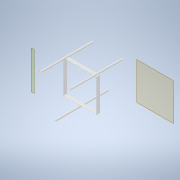
# Autodesk Inventor part: Grid
Saved by Autodesk Inventor 2020 (Build 240168000, 168)
## iProperties
Created: 2022-03-23
Part Number: Grid
Material: Genérico
Document SubType Name: Modeling
Designer: aarco
Density: 1 g/cm^3
Appearance: Valor por defecto
Mass: 1984.02 g
Surface Area: 19686.3 cm^2
Volume: 1984.02 cm^3
Author: aarco
Autodesk Inventor part; units mm, degrees
ref_plane "YZ Plane" through (0, 0, 0) normal (1, 0, 0) x (0, 1, 0)
ref_plane "XZ Plane" through (0, 0, 0) normal (0, 1, 0) x (-1, 0, 0)
ref_plane "XY Plane" through (0, 0, 0) normal (0, 0, 1) x (1, 0, 0)
ref_plane "Plano de trabajo1" through (0, 0, 0) normal (0, 0, 1) x (1, 0, 0)
ref_plane "Plano de trabajo3" through (-2370.6432, -155.0139, 1126.1413) normal (0, 0, -1) x (-1, 0, 0)
sketch "Boceto3" plane through (-2370.6432, -155.0139, 1126.1413) normal (0, 0, -1) x (-1, 0, 0)
  line L0 (-2193.4542, 373.9783) -> (-2193.4542, 1173.9783) projected
  line L1 (-1393.4542, 373.9783) -> (-2193.4542, 373.9783) projected
  line L2 (-1393.4542, 1173.9783) -> (-1393.4542, 373.9783) projected
  line L3 (-2193.4542, 1173.9783) -> (-1393.4542, 1173.9783) projected
  circle A0 centre (-1793.4542, 773.9783) radius 283.4638 projected
  line L4 (-2197.4542, 1285.9783) -> (-2237.4542, 1285.9783) construction
  line L5 (-2237.4542, 1245.9783) -> (-2237.4542, 1285.9783) construction
  line L6 (-2235.4542, 1247.9783) -> (-2235.4542, 1283.9783) projected
  line L7 (-2199.4542, 1247.9783) -> (-2235.4542, 1247.9783) projected
  line L8 (-2197.4542, 1205.9783) -> (-2197.4542, 1285.9783) construction
  line L9 (-2199.4542, 1245.9783) -> (-2235.4542, 1245.9783) construction
  line L10 (-2199.4542, 1283.9783) -> (-2199.4542, 1247.9783) projected
  line L11 (-2235.4542, 1283.9783) -> (-2199.4542, 1283.9783) projected
  line L12 (-2235.4542, 1245.9783) -> (-2237.4542, 1245.9783) construction
  line L13 (-2199.4542, 1245.9783) -> (-2197.4542, 1245.9783) construction
  line L14 (-1387.4542, 1283.9783) -> (-1351.4542, 1283.9783) projected
  line L15 (-1387.4542, 1247.9783) -> (-1387.4542, 1283.9783) projected
  line L16 (-1351.4542, 1247.9783) -> (-1387.4542, 1247.9783) projected
  line L17 (-1351.4542, 1283.9783) -> (-1351.4542, 1247.9783) projected
  line L18 (-1775.4542, 299.9783) -> (-1811.4542, 299.9783) projected
  line L19 (-1775.4542, 263.9783) -> (-1775.4542, 299.9783) projected
  line L20 (-1811.4542, 299.9783) -> (-1811.4542, 263.9783) projected
  line L21 (-1811.4542, 263.9783) -> (-1775.4542, 263.9783) projected
  line L22 (-2233.4542, 1281.9783) -> (-2201.4542, 1281.9783)
  line L23 (-2201.4542, 1281.9783) -> (-2201.4542, 1249.9783)
  line L24 (-2201.4542, 1249.9783) -> (-2233.4542, 1249.9783)
  line L25 (-2233.4542, 1249.9783) -> (-2233.4542, 1281.9783)
  line L26 (-2217.4542, 1281.9783) -> (-2217.4542, 1283.9783) construction
  line L27 (-2233.4542, 1265.9783) -> (-2235.4542, 1265.9783) construction
  line L28 (-1385.4542, 1281.9783) -> (-1353.4542, 1281.9783)
  line L29 (-1353.4542, 1281.9783) -> (-1353.4542, 1249.9783)
  line L30 (-1353.4542, 1249.9783) -> (-1385.4542, 1249.9783)
  line L31 (-1385.4542, 1249.9783) -> (-1385.4542, 1281.9783)
  line L32 (-1385.4542, 1265.9783) -> (-1387.4542, 1265.9783) construction
  line L33 (-1369.4542, 1281.9783) -> (-1369.4542, 1283.9783) construction
  line L34 (-1809.4542, 297.9783) -> (-1777.4542, 297.9783)
  line L35 (-1777.4542, 297.9783) -> (-1777.4542, 265.9783)
  line L36 (-1777.4542, 265.9783) -> (-1809.4542, 265.9783)
  line L37 (-1809.4542, 265.9783) -> (-1809.4542, 297.9783)
  line L38 (-1793.4542, 297.9783) -> (-1793.4542, 299.9783) construction
  line L39 (-1809.4542, 281.9783) -> (-1811.4542, 281.9783) construction
  line L40 (-2264.9542, 1247.9783) -> (-1321.9542, 1247.9783)
  line L41 (-1321.9542, 1247.9783) -> (-1321.9542, 304.9783)
  line L42 (-1321.9542, 304.9783) -> (-2264.9542, 304.9783)
  line L43 (-2264.9542, 304.9783) -> (-2264.9542, 1247.9783)
  line L44 (-1793.4542, 773.9783) -> (-1793.4542, 1180.8852)
  line L45 (-2262.9542, 1245.9783) -> (-1323.9542, 1245.9783)
  line L46 (-1323.9542, 1245.9783) -> (-1323.9542, 306.9783)
  line L47 (-1323.9542, 306.9783) -> (-2262.9542, 306.9783)
  line L48 (-2262.9542, 306.9783) -> (-2262.9542, 1245.9783)
  line L49 (-1793.4542, 299.9783) -> (-1793.4542, 306.9783) construction
  line L50 (-2264.9542, 776.4783) -> (-2262.9542, 776.4783)
  line L51 (-1775.4542, 299.9783) -> (-1811.4542, 299.9783)
  line L52 (-1811.4542, 299.9783) -> (-1811.4542, 304.9783)
  line L53 (-1811.4542, 304.9783) -> (-1775.4542, 304.9783)
  line L54 (-1775.4542, 304.9783) -> (-1775.4542, 299.9783)
  point P0 (-2370.6432, 155.0139)
  point P1 (-1811.4542, 299.9783)
  point P2 (-1351.4542, 1247.9783)
  point P3 (-1387.4542, 1247.9783)
  point P4 (-2199.4542, 1247.9783)
  point P5 (-2235.4542, 1247.9783)
  point P6 (515.8857, -2)
  point P7 (-1775.4542, 304.9783)
  dimension "d2" = 2
  dimension "d3" = 2
  dimension "d4" = 2
  dimension "d26" = 5
  constraints: 70 end point, 16 midpoint, 15 perpendicular, 12 parallel, 6 equal length, 6 horizontal, 3 point on line, 1 symmetric about line, 1 vertical
  measures "d2" distance of L26.start L26.end
  measures "d3" distance of L39.start L39.end
  measures "d4" distance between parallel lines of L43 L48
  measures "d26" distance of L18.end L52.end
extrude "Extrusión1" add sketch "Boceto3" along normal blind 100 contours L6 L11 L10 L7 | L7 L40 L16 L41 L42 L43 | L15 L14 L17 L16 | L42 L54 L18 L52 | L18 L19 L21 L20
sketch "Boceto4" plane through (-1048.6889, 149.9644, 1126.1413) normal (-1, 0, 0) x (0, 0, 1)
  line L0 (0, 943) -> (-100, 943) projected
  line L1 (-50, 943) -> (-50, 0)
  line L2 (0, 0) -> (-100, 0) projected
  circle A0 centre (-75, 17) radius 3.5
  circle A1 centre (-25, 17) radius 3.5
  line L3 (0, 2) -> (-100, 2) projected
  point P0 (-1126.1413, -149.9644)
  dimension "d7" = 7
  dimension "d8" = 50
  dimension "d9" = 15
  constraints: 2 centre point, 2 end point, 2 midpoint, 1 equal radius, 1 symmetric about line
  measures "d7" diameter of A0
  measures "d8" distance of A1.centre A0.centre
  measures "d9" distance from line of L3 A0.centre
extrude "Extrusión2" cut sketch "Boceto4" against normal through all
pattern_linear "Patrón rectangular1" count 19 spacing 50 along (0, 1, 0) of "Extrusión2"
sketch "Boceto6" plane through (-1048.6889, 149.9644, 1126.1413) normal (0, -1, 0) x (1, 0, 0)
  line L0 (489.5, 0) -> (453.5, 0) projected
  line L1 (489.5, -100) -> (453.5, -100) projected
  circle A0 centre (448.5, -25) radius 3.5
  circle A1 centre (448.5, -75) radius 3.5
  line L2 (453.5, 0) -> (453.5, -100) projected
  line L3 (453.5, -50) -> (-72.9896, -50) construction
  line L4 (448.5, -25) -> (448.5, -75) construction
  line L5 (453.5, 0) -> (453.5, -100) projected
  line L6 (489.5, 0) -> (489.5, -100) projected
  point P0 (1048.6889, -1126.1413)
  dimension "d15" = 50
  dimension "d16" = 7
  constraints: 4 end point, 2 centre point, 1 equal radius, 1 horizontal, 1 midpoint, 1 perpendicular, 1 symmetric about line
  measures "d15" distance of L4.start L4.end
  measures "d16" diameter of A0
extrude "Extrusión3" cut sketch "Boceto6" against normal through all contours A0 | A1
pattern_linear "Patrón rectangular2" count 8 spacing 50 along (-1, 0, 0) of "Extrusión3"
pattern_linear "Patrón rectangular3" count 9 spacing 50 along (1, 0, 0) of "Extrusión3"
sketch "Boceto7" plane through (-2370.6432, -155.0139, 1126.1413) normal (0, 0, 1) x (1, 0, 0)
  line L0 (1811.4542, 263.9783) -> (1775.4542, 263.9783) projected
  line L1 (1811.4542, 304.9783) -> (1811.4542, 263.9783) projected
  line L2 (1775.4542, 263.9783) -> (1775.4542, 304.9783) projected
  line L3 (1777.4542, 297.9783) -> (1777.4542, 265.9783) projected
  line L4 (1777.4542, 265.9783) -> (1809.4542, 265.9783) projected
  line L5 (1809.4542, 265.9783) -> (1809.4542, 297.9783) projected
  line L6 (1321.9542, 304.9783) -> (1321.9542, 1247.9783) projected
  line L7 (1775.4542, 304.9783) -> (1321.9542, 304.9783) projected
  line L8 (1775.4542, 263.9783) -> (1775.4542, 304.9783) projected
  line L9 (1811.4542, 263.9783) -> (1775.4542, 263.9783) projected
  line L10 (1811.4542, 304.9783) -> (1811.4542, 263.9783) projected
  line L11 (2264.9542, 304.9783) -> (1811.4542, 304.9783) projected
  line L12 (2264.9542, 1247.9783) -> (2264.9542, 304.9783) projected
  line L13 (2235.4542, 1247.9783) -> (2264.9542, 1247.9783) projected
  line L14 (2235.4542, 1283.9783) -> (2235.4542, 1247.9783) projected
  line L15 (2199.4542, 1283.9783) -> (2235.4542, 1283.9783) projected
  line L16 (2199.4542, 1247.9783) -> (2199.4542, 1283.9783) projected
  line L17 (1387.4542, 1247.9783) -> (2199.4542, 1247.9783) projected
  line L18 (1387.4542, 1283.9783) -> (1387.4542, 1247.9783) projected
  line L19 (1351.4542, 1283.9783) -> (1387.4542, 1283.9783) projected
  line L20 (1351.4542, 1247.9783) -> (1351.4542, 1283.9783) projected
  line L21 (1321.9542, 1247.9783) -> (1351.4542, 1247.9783) projected
  line L22 (2262.9542, 1245.9783) -> (1323.9542, 1245.9783) projected
  line L23 (2262.9542, 306.9783) -> (2262.9542, 1245.9783) projected
  line L24 (1323.9542, 306.9783) -> (2262.9542, 306.9783) projected
  line L25 (1323.9542, 1245.9783) -> (1323.9542, 306.9783) projected
  line L26 (1353.4542, 1281.9783) -> (1353.4542, 1249.9783) projected
  line L27 (1385.4542, 1281.9783) -> (1353.4542, 1281.9783) projected
  line L28 (1385.4542, 1249.9783) -> (1385.4542, 1281.9783) projected
  line L29 (1353.4542, 1249.9783) -> (1385.4542, 1249.9783) projected
  line L30 (2233.4542, 1281.9783) -> (2201.4542, 1281.9783) projected
  line L31 (2233.4542, 1249.9783) -> (2233.4542, 1281.9783) projected
  line L32 (2201.4542, 1249.9783) -> (2233.4542, 1249.9783) projected
  line L33 (2201.4542, 1281.9783) -> (2201.4542, 1249.9783) projected
  line L34 (1809.4542, 297.9783) -> (1777.4542, 297.9783) projected
  line L35 (1809.4542, 265.9783) -> (1809.4542, 297.9783) projected
  line L36 (1777.4542, 265.9783) -> (1809.4542, 265.9783) projected
  line L37 (1777.4542, 297.9783) -> (1777.4542, 265.9783) projected
  line L38 (1775.4542, 299.9783) -> (1811.4542, 299.9783)
  line L39 (1793.4542, 299.9783) -> (1793.4542, 297.9783) construction
  line L40 (1809.4542, 297.9783) -> (1777.4542, 297.9783) projected
  line L41 (1321.9542, 1247.9783) -> (1351.4542, 1247.9783) projected
  line L42 (1351.4542, 1247.9783) -> (1387.4542, 1247.9783)
  line L43 (2235.4542, 1247.9783) -> (2199.4542, 1247.9783)
  point P0 (2370.6432, 155.0139)
  point P1 (1775.4542, 299.9783)
  dimension "d30" = 2
  constraints: 8 end point, 2 horizontal, 2 midpoint, 2 point on line, 1 perpendicular
  measures "d30" distance between parallel lines of L34 L38
extrude "Extrusión4" add sketch "Boceto7" along normal blind 700 and the other way blind 800 contours L0 L2 L38 L1 | L43 L16 L15 L14 | L20 L19 L18 L42
